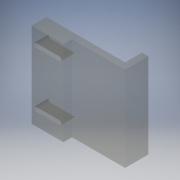
# Autodesk Inventor part: Guide
Saved by Autodesk Inventor 2019 (Build 230136000, 136)
## iProperties
Created: 2017-01-19
Part Number: Guide
Document SubType Name: Modeling
Designer: Administrator
Density: 1 g/cm^3
Mass: 7.80802 g
Surface Area: 51.034 cm^2
Volume: 7.80802 cm^3
Material: Generic
Appearance: Polycarbonate - Smoked
Author: Administrator
Autodesk Inventor part; units mm, degrees
ref_plane "YZ Plane" through (0, 0, 0) normal (1, 0, 0) x (0, 1, 0)
ref_plane "XZ Plane" through (0, 0, 0) normal (0, 1, 0) x (-1, 0, 0)
ref_plane "XY Plane" through (0, 0, 0) normal (0, 0, 1) x (1, 0, 0)
sketch "Sketch1" plane through (0, 0, 0) normal (0, 0, 1) x (1, 0, 0)
  line L0 (0, 0) -> (0, 15) construction
  line L1 (0, 15) -> (40, 15) construction
  line L2 (40, 15) -> (40, 4)
  line L3 (40, 4) -> (15, 4)
  line L4 (15, 4) -> (15, 0)
  line L5 (15, 0) -> (0, 0)
  line L6 (0, 7) -> (37, 7)
  line L7 (37, 7) -> (37, 15)
  line L8 (37, 15) -> (40, 15)
  line L9 (0, 7) -> (0, 0)
  dimension "d0" = 4
  dimension "d1" = 15
  dimension "d2" = 15
  dimension "d5" = 3
  dimension "d6" = 3
  dimension "d12" = 40
  constraints: 20 end point, 5 parallel, 2 collinear, 2 perpendicular, 2 point on line, 1 vertical, 1 other
  measures "d0" distance between parallel lines of L3 L5
  measures "d1" distance of L4.end L0.start
  measures "d2" distance between parallel lines of L1 L5
  measures "d5" distance between parallel lines of L7 L2
  measures "d6" distance between parallel lines of L6 L3
  measures "d12" distance between parallel lines of L0 L2
extrude "Extrusion1" add sketch "Sketch1" along normal blind 40
sketch "Sketch2" plane through (0, 0, 0) normal (0, -1, 0) x (1, 0, 0)
  line L0 (0, 0) -> (0, 40) projected
  line L1 (15, 0) -> (15, 40) projected
  line L2 (0, 20) -> (15, 20) construction
  line L3 (0, 33) -> (15, 33) construction
  arc A0 (2, 34) -> (2, 32) centre (2, 33) ccw
  arc A1 (13, 32) -> (13, 34) centre (13, 33) ccw
  line L4 (2, 34) -> (13, 34)
  line L5 (2, 32) -> (13, 32)
  line L6 (0, 7) -> (15, 7) construction
  arc A2 (2, 8) -> (2, 6) centre (2, 7) ccw
  arc A3 (13, 6) -> (13, 8) centre (13, 7) ccw
  line L7 (2, 6) -> (13, 6)
  line L8 (2, 8) -> (13, 8)
  dimension "d7" = 2
  dimension "d8" = 2
  dimension "d9" = 2
  dimension "d13" = 13
  constraints: 14 end point, 8 point on circle, 8 symmetric about line, 6 point on line, 4 centre point, 2 midpoint, 2 tangent, 1 equal radius, 1 parallel, 2 other
  measures "d7" diameter of A0
  measures "d8" distance from line of L0 A0.centre
  measures "d9" distance from line of A1.centre L1
  measures "d13" distance between parallel lines of L3 L2
extrude "Extrusion2" cut sketch "Sketch2" against normal blind 30
body "Solid1"
